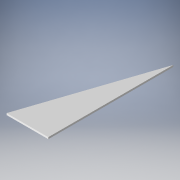
# Autodesk Inventor part: 15102898-16-P-0312
Saved by Autodesk Inventor 2017 (Build 210142000, 142)
## iProperties
Created: 2016-11-06
Part Number: 15102898-16-P-0312
Material: Generic
Document SubType Name: Modeling
Designer: gus
Density: 1 g/cm^3
Appearance: Default
Author: gus
Autodesk Inventor part; units mm, degrees
ref_plane "YZ Plane" through (0, 0, 0) normal (1, 0, 0) x (0, 1, 0)
ref_plane "XZ Plane" through (0, 0, 0) normal (0, 1, 0) x (-1, 0, 0)
ref_plane "XY Plane" through (0, 0, 0) normal (0, 0, 1) x (1, 0, 0)
sketch "Sketch1" plane through (0, 0, 0) normal (0, 1, 0) x (-1, 0, 0)
  line L0 (0, 0) -> (76.2, 152.4)
  line L1 (76.2, 152.4) -> (0, 152.4)
  line L2 (0, 152.4) -> (0, 0)
  dimension "d0" = 76.2
  dimension "d1" = 152.4
  constraints: 6 end point, 1 horizontal, 1 perpendicular
  measures "d0" distance of L0.end L1.end
  measures "d1" distance of L1.end L0.start
extrude "Extrusion1" add sketch "Sketch1" along normal blind 1.5875
sketch "Sketch2" plane through (0, 0, 0) normal (0, -1, 0) x (1, 0, 0)
  line L0 (-76.2, 152.4) -> (0, 152.4) projected
  line L1 (-74.4251, 152.4) -> (-3.175, 9.8998)
  line L2 (-3.175, 9.8998) -> (-4.5949, 9.1898)
  line L3 (0, 0) -> (-76.2, 152.4) projected
  line L4 (0, 0) -> (-76.2, 152.4) projected
  line L5 (0, 152.4) -> (0, 0) projected
  dimension "d4" = 1.5875
  dimension "d5" = 3.175
  constraints: 4 end point, 2 point on line, 1 parallel, 1 perpendicular
  measures "d4" distance between parallel lines of L3 L1
  measures "d5" distance from line of L5 L1.end
extrude "Extrusion2" add sketch "Sketch2" along normal blind 76.2 contours L0 L1 L2 L3
chamfer "Chamfer1" distance 14.2875 angle 45 1 edges at (0, 0.7937, 0)
chamfer "Chamfer2" distance 57.15 angle 63 1 edges at (-5.5958, -76.2, 12.9665)
sketch "Sketch4" plane through (-76.2, 1.5875, 152.4) normal (0, 0, 1) x (1, 0, 0)
  line L0 (0, 0) -> (1.5875, 0)
  line L1 (0, -77.7875) -> (18.2708, -77.7875) projected
  line L2 (0, -77.7875) -> (1.5875, -77.7875)
  line L3 (1.5875, -77.7875) -> (1.5875, -52.3875)
  line L4 (1.5875, -52.3875) -> (0, -52.3875)
  line L5 (0, -52.3875) -> (0, -77.7875)
  point P0 (76.2, -1.5875)
  dimension "d22" = 1.5875
  dimension "d23" = 25.4
  constraints: 10 end point, 2 horizontal, 2 parallel, 1 perpendicular
  measures "d22" distance of L4.end L3.end
  measures "d23" distance of L2.end L3.end
extrude "Extrusion4" add sketch "Sketch4" along normal blind 25.4
sketch "Sketch5" plane through (-74.6125, -76.2, 152.4) normal (1, 0, 0) x (0, 0, -1)
  line L0 (0, 0) -> (-25.4, 0) projected
  line L1 (-25.4, 25.4) -> (-25.4, 0) projected
  point P0 (152.4, 76.2)
  point P1 (-19.05, 6.35)
  dimension "d24" = 6.35
  dimension "d25" = 6.35
  measures "d24" distance from line of L0 point (-19.05, 6.35)
  measures "d25" distance from line of L1 point (-19.05, 6.35)
hole "Hole1" at (-74.6125, -69.85, 171.45) direction (-1, 0, 0) diameter 5.1594 end through all
sketch "Sketch6" plane through (-6.3896, -19.05, 12.7791) normal (-0.8944272, 0, -0.4472136) x (-0.4472136, 0, 0.8944272)
  circle A0 centre (6.35, 14.2875) radius 3.175
  line L0 (0, 20.6375) -> (156.1009, 20.6375) projected
  line L1 (0, 0) -> (0, 20.6375) projected
  point P0 (-14.2875, 19.05)
  dimension "d33" = 6.35
  dimension "d34" = 6.35
  dimension "d35" = 6.35
  constraints: 1 centre point
  measures "d33" diameter of A0
  measures "d34" distance from line of A0.centre L0
  measures "d35" distance from line of L1 A0.centre
extrude "Extrusion5" cut sketch "Sketch6" against normal blind 25.4
body "Solid1"
